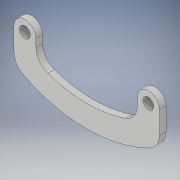
# Autodesk Inventor part: panto_linkageF
Saved by Autodesk Inventor 2017 (Build 210142000, 142)
## iProperties
Created: 2016-08-20
Part Number: panto_linkageF
Material: Generic
Document SubType Name: Modeling
Designer: Nic
Density: 1 g/cm^3
Appearance: Default
Author: Nic
Autodesk Inventor part; units mm, degrees
ref_plane "YZ Plane" through (0, 0, 0) normal (1, 0, 0) x (0, 1, 0)
ref_plane "XZ Plane" through (0, 0, 0) normal (0, 1, 0) x (-1, 0, 0)
ref_plane "XY Plane" through (0, 0, 0) normal (0, 0, 1) x (1, 0, 0)
sketch "Sketch1" plane through (0, 0, 0) normal (0, 0, 1) x (1, 0, 0)
  circle A0 centre (0, 0) radius 1.25
  line L0 (0, 0) -> (28, 0) construction
  circle A1 centre (28, 0) radius 1.25
  arc A2 (2.5, 0) -> (-2.5, 0) centre (0, 0) ccw
  arc A3 (30.5, 0) -> (25.5, 0) centre (28, 0) ccw
  line L1 (25.5, 0) -> (25.5, -1.7428)
  line L2 (30.5, 0) -> (30.5, -5.0549)
  line L3 (14, 0) -> (14, -6) construction
  arc A4 (5.1957, -5.5242) -> (22.8043, -5.5242) centre (14, 20) ccw
  arc A5 (-0.2857, -8.6342) -> (28.2857, -8.6342) centre (14, 20) ccw
  arc A6 (2.5, -1.7428) -> (5.1957, -5.5242) centre (6.5, -1.7428) ccw
  arc A7 (-2.5, -5.0549) -> (-0.2857, -8.6342) centre (1.5, -5.0549) ccw
  arc A8 (22.8043, -5.5242) -> (25.5, -1.7428) centre (21.5, -1.7428) ccw
  arc A9 (28.2857, -8.6342) -> (30.5, -5.0549) centre (26.5, -5.0549) ccw
  line L4 (-2.5, 0) -> (-2.5, -5.0549)
  line L5 (2.5, 0) -> (2.5, -1.7428)
  point P0 (30.5, -7.4181)
  point P1 (25.5, -4.4285)
  point P2 (-2.5, -7.4181)
  point P3 (2.5, -4.4285)
  dimension "d0" = 2.5
  dimension "d1" = 28
  dimension "d21" = 6
  dimension "d22" = 14
  dimension "d23" = 2.5
  dimension "d24" = 27
  dimension "d25" = 32
  dimension "d26" = 20
  dimension "d27" = 4
  constraints: 20 point on circle, 12 end point, 10 centre point, 10 tangent, 5 equal radius, 4 coincident, 4 point on line, 4 vertical, 2 symmetric about line, 1 concentric, 1 horizontal, 1 midpoint, 1 perpendicular, 1 vertical alignment
  measures "d0" diameter of A0
  measures "d1" distance of L0.start L0.end
  measures "d21" distance of L3.start L3.end
  measures "d22" distance from line of point (0, 0) L3
  measures "d23" radius of A2
  measures "d24" radius of A4
  measures "d25" radius of A5
  measures "d26" vertical distance of point (0, 0) A4.centre
  measures "d27" radius of A6
extrude "Extrusion1" add sketch "Sketch1" along normal blind 1.5
body "Solid1"
